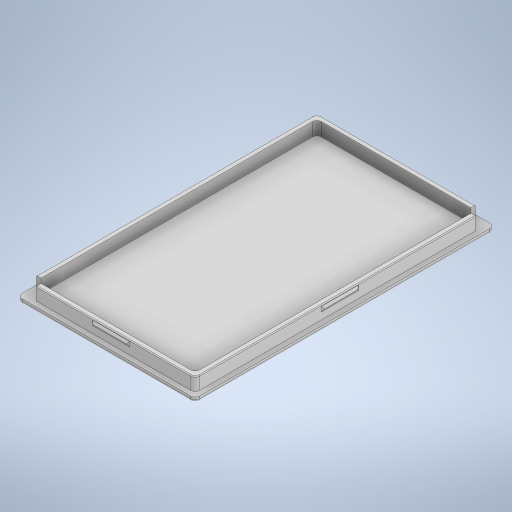
# Autodesk Inventor part: RemoteControllerBottom
Saved by Autodesk Inventor 2024 (Build 280153000, 153)
## iProperties
Created: 2025-10-14
Part Number: RemoteControllerBottom
Material: Generic
Document SubType Name: Modeling
Designer: Martin
Density: 1 g/cm^3
Appearance: Default
Author: Martin
Autodesk Inventor part; units mm, degrees
ref_plane "YZ Plane" through (0, 0, 0) normal (1, 0, 0) x (0, 1, 0)
sketch "Sketch1" plane through (0, 0, 0) normal (0, 1, 0) x (-1, 0, 0)
  line L0 (-39.9143, 68.4893) -> (74.3857, 68.4893)
  line L1 (77.5607, 65.3143) -> (77.5607, -131.5357)
  line L2 (74.3857, -134.7107) -> (-39.9143, -134.7107)
  line L3 (-43.0893, -131.5357) -> (-43.0893, 65.3143)
  arc A0 (74.3857, -134.7107) -> (77.5607, -131.5357) centre (74.3857, -131.5357) ccw
  arc A1 (-43.0893, -131.5357) -> (-39.9143, -134.7107) centre (-39.9143, -131.5357) ccw
  arc A2 (-39.9143, 68.4893) -> (-43.0893, 65.3143) centre (-39.9143, 65.3143) ccw
  arc A3 (77.5607, 65.3143) -> (74.3857, 68.4893) centre (74.3857, 65.3143) ccw
  point P0 (0, 0)
  point P1 (-43.0893, 68.4893)
  point P2 (77.5607, -134.7107)
  point P3 (77.5607, 68.4893)
  point P4 (-43.0893, -134.7107)
  dimension "d0" = 203.2
  dimension "d1" = 120.65
  dimension "d16" = 3.175
  constraints: 8 end point, 8 point on circle, 8 point on line, 8 tangent, 4 centre point, 3 equal radius, 2 parallel, 1 horizontal, 1 perpendicular
  measures "d0" distance of point (77.561, 68.489) point (77.561, -134.711)
  measures "d1" distance of point (77.561, -134.711) point (-43.089, -134.711)
  measures "d16" radius of A0
extrude "Extrusion1" add sketch "Sketch1" along normal blind 3.175
sketch "Sketch2" plane through (0, 3.175, 0) normal (0, 1, 0) x (1, 0, 0)
  line L0 (-74.3857, -68.4893) -> (39.9143, -68.4893) projected
  line L1 (-77.5607, 131.5357) -> (-77.5607, -65.3143) projected
  line L2 (39.9143, 134.7107) -> (-74.3857, 134.7107) projected
  line L3 (43.0893, -65.3143) -> (43.0893, 131.5357) projected
  line L4 (-74.2587, 128.2337) -> (-74.2587, -62.0123)
  line L5 (-71.0837, -65.1873) -> (36.6123, -65.1873)
  line L6 (39.7873, -62.0123) -> (39.7873, 128.2337)
  line L7 (36.6123, 131.4087) -> (-71.0837, 131.4087)
  line L8 (-71.0837, 125.0587) -> (-71.0837, -58.8373)
  line L9 (-67.9087, -62.0123) -> (33.4373, -62.0123)
  line L10 (36.6123, -58.8373) -> (36.6123, 125.0587)
  line L11 (33.4373, 128.2337) -> (-67.9087, 128.2337)
  arc A0 (-74.2587, -62.0123) -> (-71.0837, -65.1873) centre (-71.0837, -62.0123) ccw
  arc A1 (-71.0837, -58.8373) -> (-67.9087, -62.0123) centre (-67.9087, -58.8373) ccw
  arc A2 (33.4373, -62.0123) -> (36.6123, -58.8373) centre (33.4373, -58.8373) ccw
  arc A3 (36.6123, -65.1873) -> (39.7873, -62.0123) centre (36.6123, -62.0123) ccw
  arc A4 (39.7873, 128.2337) -> (36.6123, 131.4087) centre (36.6123, 128.2337) ccw
  arc A5 (36.6123, 125.0587) -> (33.4373, 128.2337) centre (33.4373, 125.0587) ccw
  arc A6 (-67.9087, 128.2337) -> (-71.0837, 125.0587) centre (-67.9087, 125.0587) ccw
  arc A7 (-71.0837, 131.4087) -> (-74.2587, 128.2337) centre (-71.0837, 128.2337) ccw
  line L12 (-71.0837, -58.8373) -> (-74.2587, -58.8373)
  line L13 (-67.9087, -62.0123) -> (-67.9087, -65.1873)
  line L14 (36.6123, 125.0587) -> (39.7873, 125.0587)
  line L15 (33.4373, 128.2337) -> (33.4373, 131.4087)
  point P0 (0, 0)
  point P1 (-77.5607, -68.4893)
  point P2 (43.0893, -68.4893)
  point P3 (-77.5607, 134.7107)
  point P4 (43.0893, 134.7107)
  dimension "d11" = 3.302
  dimension "d12" = 3.175
  dimension "d13" = 3.175
  constraints: 24 end point, 16 point on circle, 16 tangent, 8 centre point, 7 equal radius, 4 point on line, 3 perpendicular, 6 other
  measures "d11" distance between parallel lines of L2 L7
  measures "d12" distance between parallel lines of L7 L11
  measures "d13" radius of A0
extrude "Extrusion3" add sketch "Sketch2" along normal blind 8.89 contours A7 L7 L15 L11 A6 L8 L12 L4 | L9 A2 L10 L14 L6 A3 L5 L13
sketch "Sketch3" plane through (-74.2587, 3.175, -128.2337) normal (-1, 0, 0) x (0, 0, 1)
  line L0 (3.175, 0) -> (187.071, 0) projected
  line L1 (95.123, 0) -> (95.123, 6.4135)
  line L2 (82.423, 4.826) -> (107.823, 4.826)
  line L3 (107.823, 4.826) -> (107.823, 8.001)
  line L4 (107.823, 8.001) -> (82.423, 8.001)
  line L5 (82.423, 8.001) -> (82.423, 4.826)
  line L6 (82.423, 4.826) -> (107.823, 8.001) construction
  line L7 (107.823, 4.826) -> (82.423, 8.001) construction
  point P0 (128.2337, -3.175)
  dimension "d17" = 6.4135
  dimension "d18" = 25.4
  dimension "d19" = 3.175
  constraints: 14 end point, 3 midpoint, 2 parallel, 1 horizontal, 1 perpendicular
  measures "d17" distance of L1.start L1.end
  measures "d18" distance of L4.end L3.end
  measures "d19" distance of L2.end L3.end
extrude "Extrusion4" add sketch "Sketch3" along normal blind 8.255 draft -60
sketch "Sketch5" plane through (-67.9087, 3.175, 65.1873) normal (0, 0, 1) x (1, 0, 0)
  line L0 (0, 0) -> (0, 8.89) projected
  line L1 (101.346, 0) -> (101.346, 8.89) projected
  line L2 (63.373, 4.826) -> (37.973, 4.826)
  line L3 (37.973, 4.826) -> (37.973, 8.001)
  line L4 (37.973, 8.001) -> (63.373, 8.001)
  line L5 (63.373, 8.001) -> (63.373, 4.826)
  line L6 (63.373, 4.826) -> (37.973, 8.001) construction
  line L7 (37.973, 4.826) -> (63.373, 8.001) construction
  line L8 (-6.477, 0) -> (107.823, 0) projected
  point P0 (67.9087, -3.175)
  point P1 (50.673, 6.4135)
  dimension "d22" = 25.4
  dimension "d23" = 3.175
  dimension "d24" = 6.4135
  constraints: 12 end point, 2 midpoint, 2 parallel, 1 horizontal, 1 perpendicular
  measures "d22" distance of L3.end L4.end
  measures "d23" distance of L2.end L3.end
  measures "d24" distance from line of L8 point (50.673, 6.413)
extrude "Extrusion5" add sketch "Sketch5" along normal blind 8.89 draft -60
ref_plane "Work Plane1" through (-67.9087, 3.175, -33.1107) normal (0, 0, 1) x (1, 0, 0)
ref_plane "Work Plane2" through (-17.2357, 3.175, 62.0123) normal (1, 0, 0) x (0, 0, -1)
mirror "Mirror1" about plane through (-67.9087, 3.175, -33.1107) normal (0, 0, 1) of "Extrusion5"
mirror "Mirror2" about plane through (-17.2357, 3.175, 62.0123) normal (1, 0, 0) of "Extrusion4"
fillet "Fillet1" radius 1.5875 8 edges at (42.1594, 0, -133.7808) (-17.2357, 0, -134.7107) (-76.6308, 0, -133.7808) (-77.5607, 0, -33.1107) (-76.6308, 0, 67.5593) (-17.2357, 0, 68.4893) (42.1594, 0, 67.5593) (43.0893, 0, -33.1107)
fillet "Fillet2" radius 0.5715 6 edges at (38.8574, 12.065, 64.2573) (-15.6482, 12.065, 65.1873) (39.7873, 12.065, -31.5232) (-73.3288, 12.065, -130.4788) (-74.2587, 12.065, -34.6982) (-18.8232, 12.065, -131.4087)
body "Solid1"
